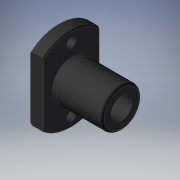
# Autodesk Inventor part: C-LHFC8
Saved by Autodesk Inventor 2019 (Build 230136000, 136)
## iProperties
Created: 2022-12-27
Part Number: C-LHFC8
Material: Generic
Catalog Web Link: www.cadenas.de
Description: C-LHFR, C-LHFS, C-LHFC, C-LHFRM, C-LHFSM, C-LHFCM-Flanged Linear Bushings - Standard - C-VALUE Single Type
Vendor: MISUMI
Document SubType Name: Modeling
Designer: psAdmin
Manufacturer: MISUMI
Mass: 5.00154 g
Surface Area: 32.0275 cm^2
Volume: 5.00154 cm^3
Density: 1 g/cm^3
Appearance: PSOLRGB-175-175-175
Category: PARTsolutions
Company: MISUMI
Title: C-LHFC8
Author: Cadenas PARTsolutions
Comments: Flanged Linear Bushings - Standard - C-VALUE Single Type
PSOL_IDENT_0: {$CADENAS_DATA/23d-libs/misumi/metric/04_linear_bushings/c_lhfr.prj},202 {VTYP=3D},{NB=C-LHFC8},{LIN
PSOL_IDENT_1: A=C-LHFC8},{NN=C-LHFR, C-LHFS, C-LHFC, C-LHFRM, C-LHFSM, C-LHFCM},{DATE=21.04.2022 04:27:33},{GEOMDA
PSOL_IDENT_2: TE=25.09.2019 05:32:57},{VERSION=},{LINEID=50},{WBVAR=TS,ST},{WBNUMERIC=}  {NB=C-LHFC8},{LINA=C-LHFC
PSOL_IDENT_3: 8},{KT=DUMMY},{PN=C-LHFC8},{TYPE=C-LHFC},{TS=C},{TSALG='R', 'Round Flange', 'S', 'Square Flange', 'C'
PSOL_IDENT_4: , '2 - Flats Flange'},{ST=},{DDRR=8},{D=15},{L=24},{H=32},{T=5},{DD=3.5},{DD1=6.0},{TT=3.1},{PCD=0},
PSOL_IDENT_5: {PCDFX=24},{W=0},{WFX=25},{F=0},{FFX=0},{A=24},{AFX=24},{BR=4},{TIFF=3},{R=0.9}
NB: C-LHFC8
NN: C-LHFR, C-LHFS, C-LHFC, C-LHFRM, C-LHFSM, C-LHFCM
NT: Flanged Linear Bushings - Standard - C-VALUE Single Type
NBSYN: $PN.
LINA: C-LHFC8
CATALOG: Misumi
PN: C-LHFC8
TS: 2 - Flats Flange
ST: -
DDRR: 8
D: 15
L: 24
H: 32
T: 5
DD: 3.5
DD1: 6
TT: 3.1
PCD: 0
W: 0
F: 0
A: 24
SUPPLIER: MISUMI
ARTICLENO: C-LHFC8
BOMINFO: C-LHFC8
CREATOR: CADENAS GmbH
Autodesk Inventor part; units mm, degrees
sketch "Sketch_1" plane through (0, 0, 0) normal (0, 0, 1) x (1, 0, 0)
  line L0 (24, 0) -> (0, 0)
  line L1 (0, 4) -> (24, 4)
  line L2 (24, 4) -> (24, 6.6)
  arc A0 (24, 6.6) -> (23.1, 7.5) centre (23.1, 6.6) ccw
  line L3 (23.1, 7.5) -> (6.6, 7.5)
  line L4 (6.6, 7.5) -> (6.6, 7.25)
  line L5 (6.6, 7.25) -> (5, 7.25)
  line L6 (5, 7.25) -> (5, 15.5)
  line L7 (5, 15.5) -> (4.5, 16)
  line L8 (4.5, 16) -> (0.5, 16)
  line L9 (0.5, 16) -> (0, 15.5)
  line L10 (0, 15.5) -> (0, 4)
  constraints: 22 end point, 2 point on circle, 1 centre point
revolve "Revolution1" add sketch "Sketch_1" angle 360 about axis through (24, 0, 0) along (1, 0, 0)
sketch "Sketch_3" plane through (0, 0, 0) normal (1, 0, 0) x (0, 1, 0)
  line L0 (-32, 32) -> (-32, -32)
  line L1 (-32, -32) -> (32, -32)
  line L2 (32, -32) -> (32, 32)
  line L3 (32, 32) -> (-32, 32)
  line L4 (12.0727, 10.5) -> (-12.0727, 10.5)
  arc A0 (-12.0727, 10.5) -> (-12.0727, -10.5) centre (0, 0) ccw
  line L5 (-12.0727, -10.5) -> (12.0727, -10.5)
  arc A1 (12.0727, -10.5) -> (12.0727, 10.5) centre (0, 0) ccw
  constraints: 12 end point, 4 point on circle, 2 centre point
extrude "Extrusion1" cut sketch "Sketch_3" along normal blind 5
sketch "Sketch3" plane through (0, -11.4018, -10.5) normal (-1, 0, 0) x (0, 0, 1)
  point P0 (10.5, 23.4018)
hole "Hole1" at (0, 12, 0) direction (1, 0, 0) diameter 3.5 depth 5 counterbore diameter 6 counterbore depth 3.1
sketch "Sketch4" plane through (0, -11.4018, -10.5) normal (-1, 0, 0) x (0, 0, 1)
  point P0 (10.5, -0.5982)
hole "Hole2" at (0, -12, 0) direction (1, 0, 0) diameter 3.5 depth 5 counterbore diameter 6 counterbore depth 3.1
ref_plane "Combination_Module_XY" through (0, 0, 0) normal (1, 0, 0) x (0, 0, -1)
ref_plane "Combination_Module_YZ" through (0, 0, 0) normal (0, 0, -1) x (0, 1, 0)
ref_plane "Combination_Module_ZX" through (0, 0, 0) normal (0, 1, 0) x (1, 0, 0)
body "Solid1"
